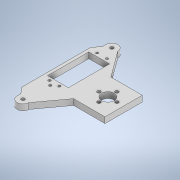
# Autodesk Inventor part: Claw_Main
Saved by Autodesk Inventor 2022 (Build 260153000, 153)
## iProperties
Created: 2022-03-18
Part Number: Claw_Main
Material: Generic
Document SubType Name: Modeling
Designer: Mlees
Density: 1 g/cm^3
Appearance: Default
Author: Mlees
Autodesk Inventor part; units mm, degrees
ref_plane "YZ Plane" through (0, 0, 0) normal (1, 0, 0) x (0, 1, 0)
ref_plane "XZ Plane" through (0, 0, 0) normal (0, 1, 0) x (-1, 0, 0)
ref_plane "XY Plane" through (0, 0, 0) normal (0, 0, 1) x (1, 0, 0)
sketch "Sketch1" plane through (0, 0, 0) normal (0, 1, 0) x (-1, 0, 0)
  line L0 (0, 0) -> (0, -19)
  line L1 (0, 0) -> (0, 19)
  line L2 (0, 0) -> (19, 0) construction
  line L3 (0, 19) -> (32, 19)
  line L4 (0, -19) -> (32, -19)
  line L5 (68.5, 0) -> (68.5, -35)
  line L6 (68.5, 0) -> (68.5, 35)
  circle A0 centre (16, 0) radius 6.5
  circle A1 centre (25.125, 0) radius 1.75
  line L7 (55, -30) -> (44.25, -30)
  line L8 (44.25, -30) -> (44.25, 12)
  line L9 (44.25, 12) -> (65.5, 12)
  line L10 (65.5, 12) -> (65.5, 0)
  line L11 (65.5, 0) -> (65.5, -30)
  line L12 (65.5, -30) -> (55, -30)
  line L13 (68.5, -30) -> (68.5, -32)
  circle A2 centre (60.25, -33.25) radius 1.25
  circle A3 centre (50.25, -33.25) radius 1.25
  circle A4 centre (60.25, 15.25) radius 1.25
  circle A5 centre (50.25, 15.25) radius 1.25
  circle A6 centre (16, 9.125) radius 1.75
  circle A7 centre (6.875, 0) radius 1.75
  circle A8 centre (16, -9.125) radius 1.75
  line L14 (68.5, 0) -> (65.5, 0)
  circle A9 centre (57.25, -45.25) radius 1.75
  line L15 (55.5, -45.25) -> (49.3011, -45.25)
  arc A10 (51.25, -45.25) -> (63.25, -45.25) centre (57.25, -45.25) ccw
  line L16 (51.25, -45.25) -> (32, -19)
  line L17 (63.25, -41.5) -> (63.25, -45.25)
  line L18 (68.5, -35) -> (63.25, -41.5)
  circle A11 centre (57.25, 45.25) radius 1.75
  arc A12 (63.25, 45.25) -> (51.25, 45.25) centre (57.25, 45.25) ccw
  line L19 (51.25, 45.25) -> (32, 19)
  line L20 (63.25, 41.5) -> (63.25, 45.25)
  line L21 (68.5, 35) -> (63.25, 41.5)
  circle A13 centre (55.5, 19.25) radius 1.25
  dimension "d0" = 19
  dimension "d1" = 19
  dimension "d2" = 90
  dimension "d3" = 32
  dimension "d4" = 68.5
  dimension "d5" = 35
  dimension "d8" = 13
  dimension "d10" = 3.5
  dimension "d18" = 10.75
  dimension "d22" = 2.5
  dimension "d30" = 360
  dimension "d35" = 12
  constraints: 44 end point, 13 centre point, 6 perpendicular, 5 symmetric about line, 4 point on circle, 4 vertical, 3 horizontal, 2 coincident, 1 horizontal alignment, 1 point on line, 1 tangent, 13 other
  measures "d0" distance of L0.start L0.end
  measures "d1" distance of L0.start L1.end
  measures "d2" angle of L2 L1
  measures "d3" distance of L1.end L3.end
  measures "d4" distance of L0.start L5.start
  measures "d5" distance of L5.start L5.end
  measures "d8" diameter of A0
  measures "d10" diameter of A1
  measures "d18" distance of L7.start L7.end
  measures "d22" diameter of A2
  measures "d35" diameter of A10
extrude "Extrusion1" add sketch "Sketch1" along normal blind 6
body "Solid1"
